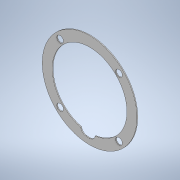
# Autodesk Inventor part: 75. Прокладка крышки
Saved by Autodesk Inventor 2021 (Build 250183000, 183)
## iProperties
Created: 2021-03-11
Part Number: 75. Прокладка крышки
Material: Типовые
Document SubType Name: Modeling
Designer: Данил
Density: 1 g/cm^3
Appearance: По умолчанию
Author: Данил
Autodesk Inventor part; units mm, degrees
ref_plane "YZ Plane" through (0, 0, 0) normal (1, 0, 0) x (0, 1, 0)
ref_plane "XZ Plane" through (0, 0, 0) normal (0, 1, 0) x (-1, 0, 0)
ref_plane "XY Plane" through (0, 0, 0) normal (0, 0, 1) x (1, 0, 0)
sketch "Эскиз1" plane through (0, 0, 0) normal (0, 0, 1) x (1, 0, 0)
  circle A0 centre (0, 0) radius 58
  arc A1 (6.8914, -45.228) -> (-10.8071, -44.4552) centre (0, 0) ccw
  circle A2 centre (0, 0) radius 51 construction
  circle A3 centre (36.0624, 36.0624) radius 4.05
  circle A4 centre (-36.0624, 36.0624) radius 4.05
  circle A5 centre (-36.0624, -36.0624) radius 4.05
  circle A6 centre (36.0624, -36.0624) radius 4.05
  line L0 (0, 0) -> (0, 51) construction
  line L1 (0, 0) -> (36.0624, 36.0624) construction
  line L2 (0, 0) -> (-36.0624, 36.0624) construction
  line L3 (0, 0) -> (36.0624, -36.0624) construction
  line L4 (0, 0) -> (-36.0624, -36.0624) construction
  line L5 (0, 0) -> (0, -51) construction
  line L6 (0, 0) -> (-4.4449, -50.8059) construction
  arc A7 (-10.8071, -44.4552) -> (-4.4449, -50.8059) centre (-3.8349, -43.8326) ccw
  arc A8 (0, -51) -> (6.8914, -45.228) centre (0, -44) ccw
  arc A9 (-4.4449, -50.8059) -> (0, -51) centre (0, 0) ccw
  dimension "d2" = 102
  dimension "d0" = 116
  dimension "d1" = 91.5
  dimension "d3" = 8.1
  dimension "d4" = 45
  dimension "d5" = 90
  dimension "d6" = 90
  dimension "d7" = 45
  dimension "d8" = 5
  dimension "d9" = 7
  dimension "d10" = 7
  constraints: 14 end point, 9 centre point, 8 point on circle, 4 coincident, 3 equal radius, 2 point on line, 1 vertical, 1 vertical alignment, 12 other
  measures "d0" diameter of A0
  measures "d1" diameter of A1
  measures "d3" diameter of A3
  measures "d4" angle of L1 L0
  measures "d5" angle of L3 L1
  measures "d6" angle of L4 L3
  measures "d7" angle of L2 L0
  measures "d8" angle of L6 L5
  measures "d9" radius of A7
  measures "d10" radius of A8
extrude "Выдавливание1" add sketch "Эскиз1" along normal mid plane 1
